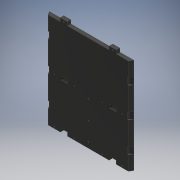
# Autodesk Inventor part: BA04
Saved by Autodesk Inventor 2017 (Build 210142000, 142)
## iProperties
Created: 2019-05-22
Part Number: BA04
Material: Wood (Cherry)
Document SubType Name: Modeling
Designer: Dell
Density: 0.63 g/cm^3
Appearance: Smooth - Black
Mass: 812.03 g
Surface Area: 2237.73 cm^2
Volume: 1288.94 cm^3
Author: Dell
Autodesk Inventor part; units mm, degrees
ref_plane "YZ Plane" through (0, 0, 0) normal (1, 0, 0) x (0, 1, 0)
ref_plane "XZ Plane" through (0, 0, 0) normal (0, 1, 0) x (-1, 0, 0)
ref_plane "XY Plane" through (0, 0, 0) normal (0, 0, 1) x (1, 0, 0)
sketch "Sketch1" plane through (0, 0, 0) normal (0, 0, 1) x (1, 0, 0)
  line L0 (0, 0) -> (303.5592, 0)
  line L1 (303.5592, 0) -> (455.3388, -262.89) construction
  line L2 (455.3388, -262.89) -> (404.5388, -350.8782)
  line L3 (404.5388, -350.8782) -> (-50.8, -87.9882) construction
  line L4 (-50.8, -87.9882) -> (0, 0) construction
  line L5 (0, 0) -> (7.3323, -12.7)
  line L6 (7.3323, -12.7) -> (296.2269, -12.7)
  line L7 (296.2269, -12.7) -> (303.5592, 0)
  dimension "d0" = 525.78
  dimension "d1" = 101.6
  dimension "d2" = 120
  dimension "d3" = 12.7
  dimension "d4" = 60
  dimension "d5" = 60
  constraints: 16 end point, 2 equal length, 2 horizontal, 2 perpendicular
  measures "d0" distance of L2.end L3.end
  measures "d1" distance of L3.end L0.start
  measures "d2" angle of L0 L4
  measures "d3" distance between parallel lines of L0 L6
  measures "d4" angle of L0 L5
  measures "d5" angle of L0 L7
extrude "Extrusion1" add sketch "Sketch1" along normal blind 342.9
sketch "Sketch2" plane through (7.3323, -12.7, 0) normal (0, -1, 0) x (1, 0, 0)
  line L0 (296.2269, 342.9) -> (-7.3323, 342.9) projected
  line L1 (43.4677, 342.9) -> (68.8677, 342.9)
  line L2 (68.8677, 342.9) -> (68.8677, 355.6)
  line L3 (68.8677, 355.6) -> (43.4677, 355.6)
  line L4 (43.4677, 355.6) -> (43.4677, 342.9)
  line L5 (220.0269, 342.9) -> (245.4269, 342.9)
  line L6 (245.4269, 342.9) -> (245.4269, 355.6)
  line L7 (245.4269, 355.6) -> (220.0269, 355.6)
  line L8 (220.0269, 355.6) -> (220.0269, 342.9)
  line L9 (-7.3323, 0) -> (-7.3323, 342.9) projected
  line L10 (296.2269, 0) -> (296.2269, 342.9) projected
  circle A0 centre (56.1677, 349.25) radius 2.25
  circle A1 centre (232.7269, 349.25) radius 2.25
  point P0 (56.1677, 355.6)
  point P1 (232.7269, 355.6)
  point P2 (68.8677, 349.25)
  point P3 (245.4269, 349.25)
  dimension "d8" = 25.4
  dimension "d9" = 12.7
  dimension "d10" = 25.4
  dimension "d11" = 12.7
  dimension "d12" = 50.8
  dimension "d13" = 50.8
  dimension "d16" = 4.5
  dimension "d17" = 4.5
  constraints: 16 end point, 4 midpoint, 4 parallel, 2 centre point, 2 horizontal, 2 horizontal alignment, 2 perpendicular, 2 point on line, 2 vertical alignment
  measures "d8" distance of L3.end L2.end
  measures "d9" distance of L2.end L1.end
  measures "d10" distance of L7.end L6.end
  measures "d11" distance of L6.end L5.end
  measures "d12" distance between parallel lines of L9 L4
  measures "d13" distance between parallel lines of L10 L6
  measures "d16" diameter of A0
  measures "d17" diameter of A1
extrude "Extrusion2" add sketch "Sketch2" against normal blind 12.7
ref_plane "Work Plane1" through (0, 0, 292.1) normal (0, 0, 1) x (1, 0, 0)
sketch "Sketch3" plane through (0, 0, 292.1) normal (0, 0, 1) x (1, 0, 0)
  line L0 (0, 0) -> (303.5592, 0) projected
  line L1 (0, 0) -> (0, -12.7)
  line L2 (296.2269, -12.7) -> (7.3323, -12.7) projected
  line L3 (0, -12.7) -> (7.3323, -12.7)
  line L4 (7.3323, -12.7) -> (0, 0) projected
  constraints: 4 end point, 1 perpendicular, 1 vertical
extrude "Extrusion3" add sketch "Sketch3" against normal blind 25.4
ref_plane "Work Plane2" through (0, 0, 50.8) normal (0, 0, -1) x (-1, 0, 0)
sketch "Sketch4" plane through (0, 0, 50.8) normal (0, 0, -1) x (-1, 0, 0)
  line L0 (0, -12.7) -> (0, 0) projected
  line L1 (-7.3323, -12.7) -> (0, 0) projected
  line L2 (-7.3323, -12.7) -> (0, -12.7) projected
extrude "Extrusion4" add sketch "Sketch4" against normal blind 25.4
ref_plane "Work Plane3" through (0, 0, 171.45) normal (0, 0, -1) x (-1, 0, 0)
sketch "Sketch5" plane through (0, 0, 171.45) normal (0, 0, -1) x (-1, 0, 0)
  line L0 (0, 0) -> (0, -12.7) projected
  line L1 (0, -12.7) -> (-7.3323, -12.7) projected
  line L2 (0, 0) -> (-7.3323, -12.7) projected
extrude "Extrusion5" add sketch "Sketch5" along normal mid plane 25.4
ref_plane "Work Plane4" through (151.7796, -12.7, 342.9) normal (-1, 0, 0) x (0, 0, 1)
mirror "Mirror1" about plane through (151.7796, -12.7, 342.9) normal (-1, 0, 0) of "Extrusion5", "Extrusion4", "Extrusion3"
sketch "Sketch6" plane through (296.2269, -12.7, 292.1) normal (0, 0, 1) x (1, 0, 0)
  line L0 (0, 0) -> (7.3323, 12.7) projected
  line L1 (7.3323, 0) -> (0, 0) projected
  line L2 (7.3323, 12.7) -> (7.3323, 0) projected
  line L3 (7.3323, 12.7) -> (7.3323, 0) projected
  line L4 (0, 0) -> (7.3323, 12.7) projected
  line L5 (7.3323, 0) -> (0, 0) projected
  line L6 (-296.2269, 12.7) -> (-296.2269, 0) projected
  line L7 (-296.2269, 0) -> (-288.8945, 0) projected
  line L8 (-296.2269, 12.7) -> (-288.8945, 0) projected
  line L9 (-296.2269, 0) -> (-296.2269, 12.7) projected
  line L10 (-296.2269, 12.7) -> (-274.2298, 0) construction
  line L11 (0, 0) -> (-288.8945, 0) projected
  line L12 (-285.2269, 6.3491) -> (-285.2269, 0)
  line L13 (-288.8945, 0) -> (-296.2269, 0) projected
  line L14 (-285.2269, 0) -> (-296.2269, 0)
  line L15 (-144.4473, 0) -> (-144.4473, -42.8761)
  line L16 (7.3323, 12.7) -> (7.3323, 0)
  line L17 (7.3323, 0) -> (0, 0)
  line L18 (7.3323, 12.7) -> (0, 0)
  line L19 (7.3323, 0) -> (7.3323, 12.7)
  line L20 (7.3323, 12.7) -> (-14.6647, 0) construction
  line L21 (-3.6677, 6.3491) -> (-3.6677, 0)
  line L22 (0, 0) -> (7.3323, 0)
  line L23 (-3.6677, 0) -> (7.3323, 0)
  line L24 (-288.8945, 0) -> (-296.2269, 12.7) projected
  line L25 (-285.2269, 6.3491) -> (-296.2269, 12.7)
  line L26 (7.3323, 12.7) -> (0, 0) projected
  line L27 (7.3323, 12.7) -> (-3.6677, 6.3491)
  line L28 (0, 0) -> (7.3323, 12.7)
  line L29 (0, 0) -> (-3.6677, 0)
  line L30 (7.3323, 0) -> (7.3323, 12.7) projected
  line L31 (-3.6677, 0) -> (7.3323, 0)
  dimension "d26" = 60
  dimension "d27" = 11
  constraints: 34 end point, 5 symmetric about line, 3 point on line, 2 collinear, 2 horizontal, 1 midpoint, 1 perpendicular, 1 vertical
  measures "d26" angle of L6 L10
  measures "d27" distance between parallel lines of L6 L12
extrude "Extrusion6" cut sketch "Sketch6" against normal blind 25.4
sketch "Sketch7" plane through (0, 0, 184.15) normal (0, 0, 1) x (1, 0, 0)
  line L0 (7.3323, -12.7) -> (0, 0) projected
  line L1 (11, -12.7) -> (7.3323, -12.7) projected
  line L2 (11, -6.3509) -> (11, -12.7) projected
  line L3 (0, 0) -> (11, -6.3509) projected
  line L4 (303.5592, 0) -> (296.2269, -12.7) projected
  line L5 (292.5592, -6.3509) -> (303.5592, 0) projected
  line L6 (292.5592, -12.7) -> (292.5592, -6.3509) projected
  line L7 (296.2269, -12.7) -> (292.5592, -12.7) projected
  line L8 (303.5592, 0) -> (303.5592, -12.7) projected
  line L9 (296.2269, -12.7) -> (303.5592, 0) projected
  line L10 (303.5592, -12.7) -> (296.2269, -12.7) projected
  line L11 (0, 0) -> (0, -12.7) projected
  line L12 (0, -12.7) -> (7.3323, -12.7) projected
  line L13 (0, 0) -> (7.3323, -12.7) projected
extrude "Extrusion7" cut sketch "Sketch7" against normal blind 25.4
sketch "Sketch8" plane through (0, 0, 76.2) normal (0, 0, 1) x (1, 0, 0)
  line L0 (0, 0) -> (0, -12.7) projected
  line L1 (0, -12.7) -> (7.3323, -12.7) projected
  line L2 (0, 0) -> (7.3323, -12.7) projected
  line L3 (7.3323, -12.7) -> (0, 0) projected
  line L4 (11, -12.7) -> (7.3323, -12.7) projected
  line L5 (11, -6.3509) -> (11, -12.7) projected
  line L6 (0, 0) -> (11, -6.3509) projected
  line L7 (303.5592, 0) -> (296.2269, -12.7) projected
  line L8 (292.5592, -6.3509) -> (303.5592, 0) projected
  line L9 (292.5592, -12.7) -> (292.5592, -6.3509) projected
  line L10 (296.2269, -12.7) -> (292.5592, -12.7) projected
  line L11 (303.5592, 0) -> (303.5592, -12.7) projected
  line L12 (296.2269, -12.7) -> (303.5592, 0) projected
  line L13 (303.5592, -12.7) -> (296.2269, -12.7) projected
extrude "Extrusion8" cut sketch "Sketch8" against normal blind 25.4
sketch "Sketch9" plane through (0, 0, 0) normal (0, 0, -1) x (-1, 0, 0)
  line L0 (-251.9796, -12.7) -> (-251.9796, 0)
  line L1 (-251.9796, 0) -> (-226.5796, 0)
  line L2 (-226.5796, 0) -> (-226.5796, -12.7)
  line L3 (-226.5796, -12.7) -> (-251.9796, -12.7)
  line L4 (-76.9796, -12.7) -> (-76.9796, 0)
  line L5 (-76.9796, 0) -> (-51.5796, 0)
  line L6 (-51.5796, 0) -> (-51.5796, -12.7)
  line L7 (-51.5796, -12.7) -> (-76.9796, -12.7)
  line L8 (-239.2796, 0) -> (-64.2796, 0) construction
  circle A0 centre (-239.2796, -6.35) radius 2.25
  circle A1 centre (-64.2796, -6.35) radius 2.25
  line L9 (-239.2796, -6.35) -> (-239.2796, 0) construction
  line L10 (-239.2796, -6.35) -> (-226.5796, -6.35) construction
  line L11 (-76.9796, -6.35) -> (-64.2796, -6.35) construction
  line L12 (-64.2796, -6.35) -> (-64.2796, 0) construction
  line L13 (0, 0) -> (-303.5592, 0) projected
  point P0 (-151.7796, 0)
  dimension "d34" = 25.4
  dimension "d35" = 12.7
  dimension "d36" = 12.7
  dimension "d37" = 25.4
  dimension "d38" = 175
  dimension "d39" = 4.5
  dimension "d40" = 4.5
  constraints: 26 end point, 6 midpoint, 6 perpendicular, 4 parallel, 4 point on line, 2 centre point
  measures "d34" distance of L4.end L5.end
  measures "d35" distance of L5.end L7.start
  measures "d36" distance of L0.start L1.start
  measures "d37" distance of L1.start L2.start
  measures "d38" distance of L8.start L12.end
  measures "d39" diameter of A0
  measures "d40" diameter of A1
extrude "Extrusion9" cut sketch "Sketch9" against normal blind 12.7 contours L0 L1 L2 L3 | L4 L5 L6 L7 | A0 | A1
sketch "Sketch10" plane through (227.3592, -12.7, 355.6) normal (0, -1, 0) x (1, 0, 0)
  line L0 (-175.7796, -194.15) -> (-150.3796, -194.15)
  line L1 (-150.3796, -194.15) -> (-150.3796, -181.45)
  line L2 (-150.3796, -181.45) -> (-175.7796, -181.45)
  line L3 (-175.7796, -181.45) -> (-175.7796, -194.15)
  line L4 (-0.7796, -194.15) -> (24.6204, -194.15)
  line L5 (24.6204, -194.15) -> (24.6204, -181.45)
  line L6 (24.6204, -181.45) -> (-0.7796, -181.45)
  line L7 (-0.7796, -181.45) -> (-0.7796, -194.15)
  line L8 (-175.7796, -342.9) -> (-150.3796, -342.9) projected
  line L9 (-0.7796, -342.9) -> (24.6204, -342.9) projected
  line L10 (-220.0269, -171.45) -> (-216.3592, -171.45) projected
  point P0 (-227.3592, -355.6)
  point P1 (-163.0796, -194.15)
  point P2 (-163.0796, -342.9)
  point P3 (11.9204, -194.15)
  point P4 (11.9204, -342.9)
  dimension "d44" = 25.4
  dimension "d45" = 12.7
  dimension "d46" = 25.4
  dimension "d47" = 12.7
  dimension "d48" = 10
  constraints: 16 end point, 4 midpoint, 4 parallel, 2 horizontal, 2 perpendicular, 2 vertical alignment, 1 horizontal alignment
  measures "d44" distance of L2.end L1.end
  measures "d45" distance of L1.end L0.end
  measures "d46" distance of L6.end L5.end
  measures "d47" distance of L5.end L4.end
  measures "d48" distance between parallel lines of L10 L2
extrude "Extrusion10" cut sketch "Sketch10" against normal through all
sketch "Sketch11" plane through (227.3592, -12.7, 355.6) normal (0, -1, 0) x (1, 0, 0)
  line L0 (-150.3796, -355.6) -> (-0.7796, -355.6) construction
  line L1 (-100.9796, -355.6) -> (-50.1796, -355.6) construction
  line L2 (-50.1796, -355.6) -> (-50.1796, -181.45) construction
  line L3 (-50.1796, -181.45) -> (-100.9796, -181.45) construction
  line L4 (-100.9796, -181.45) -> (-100.9796, -355.6) construction
  circle A0 centre (-75.5796, -268.525) radius 4
  circle A1 centre (-75.5796, -201.45) radius 4
  circle A2 centre (-75.5796, -335.6) radius 4
  line L5 (-0.7796, -355.6) -> (-150.3796, -355.6) projected
  circle A3 centre (-197.9032, -187.8) radius 2.25
  circle A4 centre (-197.9032, -349.25) radius 2.25
  circle A5 centre (46.744, -349.25) radius 2.25
  circle A6 centre (46.744, -187.8) radius 2.25
  line L6 (-175.7796, -355.6) -> (-220.0269, -355.6) projected
  line L7 (68.8677, -355.6) -> (24.6204, -355.6) projected
  line L8 (-175.7796, -194.15) -> (-175.7796, -181.45) projected
  line L9 (-175.7796, -355.6) -> (-175.7796, -342.9) projected
  line L10 (24.6204, -342.9) -> (24.6204, -355.6) projected
  line L11 (24.6204, -181.45) -> (24.6204, -194.15) projected
  circle A7 centre (-126.3796, -187.8) radius 2.25
  circle A8 centre (-126.3796, -349.25) radius 2.25
  circle A9 centre (-24.7796, -349.25) radius 2.25
  circle A10 centre (-24.7796, -187.8) radius 2.25
  point P0 (-227.3592, -355.6)
  point P1 (-150.3796, -181.45)
  point P2 (-75.5796, -355.6)
  point P3 (-75.5796, -355.6)
  point P4 (-75.5796, -355.6)
  point P5 (-50.1796, -268.525)
  point P6 (-197.9032, -355.6)
  point P7 (46.744, -355.6)
  point P8 (-175.7796, -187.8)
  point P9 (-175.7796, -349.25)
  point P10 (24.6204, -349.25)
  point P11 (24.6204, -187.8)
  point P12 (24.6204, -349.25)
  dimension "d52" = 8
  dimension "d53" = 8
  dimension "d54" = 8
  dimension "d55" = 20
  dimension "d56" = 20
  dimension "d59" = 50.8
  dimension "d60" = 4.5
  dimension "d61" = 4.5
  dimension "d62" = 4.5
  dimension "d63" = 4.5
  dimension "d64" = 4.5
  dimension "d65" = 4.5
  dimension "d66" = 4.5
  dimension "d67" = 4.5
  dimension "d68" = 25.4
  dimension "d69" = 25.4
  constraints: 11 centre point, 11 midpoint, 10 horizontal alignment, 9 vertical alignment, 8 end point, 2 parallel, 1 coincident, 1 horizontal, 1 perpendicular, 1 point on line
  measures "d52" diameter of A0
  measures "d53" diameter of A1
  measures "d54" diameter of A2
  measures "d55" distance from line of L3 A1.centre
  measures "d56" distance from line of L0 A2.centre
  measures "d59" distance of L2.end L3.end
  measures "d60" diameter of A3
  measures "d61" diameter of A4
  measures "d62" diameter of A5
  measures "d63" diameter of A6
  measures "d64" diameter of A7
  measures "d65" diameter of A8
  measures "d66" diameter of A9
  measures "d67" diameter of A10
  measures "d68" distance from line of L2 A10.centre
  measures "d69" distance from line of A7.centre L4
extrude "Extrusion11" cut sketch "Sketch11" against normal through all
equation "\"d35\" = d41"
equation "\"d36\" = d41"
equation "\"d41\" = 12.7"
body "Solid1"
